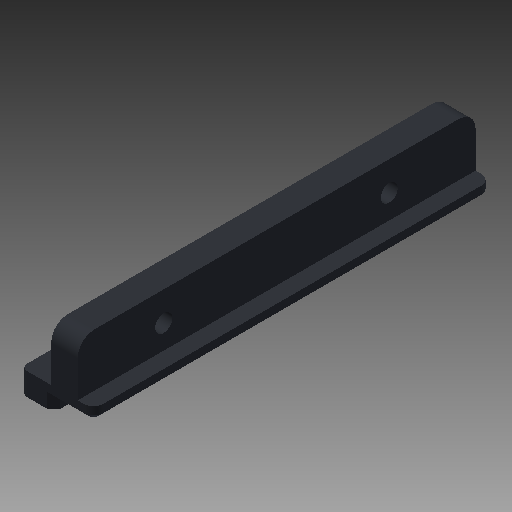
# Autodesk Inventor part: J007812
Saved by Autodesk Inventor 2018.3 (Build 223284000, 284)
## iProperties
Created: 2015-12-21
Material: VERO BLACK
Vendor: HHMI: JRC - ID&F
Document SubType Name: Modeling
Designer: ARNOLDJ
Density: 1.17 g/cm^3
Appearance: Black Anodize
Mass: 8.45789 g
Surface Area: 45.9199 cm^2
Volume: 7.22896 cm^3
Description: NRB LOW GUIDE RAIL INSERTS
Project: COMMON
Part Number: J007812
RuleStatus: InUse
AfterDocSave0: file://Part Number Cleaner
LAB/DEPT: COMMON
REQUESTING SCIENTIST: COMMON
SURFACE ROUGHNESS: N/A
DESIGN DEPARTMENT: HHMI: JRC - ID&F
SPECIAL FINISH: NONE
ALTERED ITEM PART NUMBER: N/A
ALTERED ITEM VENDOR: N/A
ALTERED ITEM DESCRIPTION: N/A
Revision Number: 0
Autodesk Inventor part; units mm, degrees
ref_plane "YZ Plane" through (0, 0, 0) normal (1, 0, 0) x (0, 1, 0)
ref_plane "XZ Plane" through (0, 0, 0) normal (0, 1, 0) x (-1, 0, 0)
ref_plane "XY Plane" through (0, 0, 0) normal (0, 0, 1) x (1, 0, 0)
sketch "Sketch1" plane through (0, 0, 0) normal (0, 0, 1) x (1, 0, 0)
  line L0 (0, 17.3736) -> (0, -2.8956) projected
  line L1 (-5.334, 0) -> (14.224, 0) projected
  line L2 (3.81, 1.778) -> (-2.54, 1.778)
  line L3 (-2.54, 1.778) -> (-2.54, 0)
  line L4 (-2.54, 0) -> (3.81, 0)
  line L5 (3.81, 0) -> (3.81, 1.778)
  line L6 (3.81, 1.778) -> (11.43, 1.778)
  line L7 (11.43, 1.778) -> (11.43, 4.318)
  line L8 (11.43, 4.318) -> (-2.54, 4.318)
  line L9 (-2.54, 4.318) -> (-2.54, 1.778)
  line L10 (8.382, 4.318) -> (3.302, 4.318)
  line L11 (3.302, 4.318) -> (3.302, 14.478)
  line L12 (3.302, 14.478) -> (8.382, 14.478)
  line L13 (8.382, 14.478) -> (8.382, 4.318)
  point P0 (0, 0)
  point P1 (0, 0.635)
  dimension "d1" = 2.54
  dimension "d2" = 1.778
  dimension "d25" = 2.54
  dimension "d26" = 10.16
  dimension "d27" = 5.08
  dimension "d49" = 3.302
  dimension "d50" = 2.54
  dimension "d51" = 11.43
  dimension "d52" = 3.81
  constraints: 24 end point, 5 perpendicular, 4 parallel, 3 horizontal, 3 point on line
  measures "d1" distance of L6.end L7.end
  measures "d2" distance of L4.end L2.start
  measures "d25" distance between parallel lines of L3 L0
  measures "d26" distance of L12.end L10.start
  measures "d27" distance of L11.end L12.end
  measures "d49" distance between parallel lines of L0 L11
  measures "d50" distance between parallel lines of L0 L9
  measures "d51" distance between parallel lines of L7 L0
  measures "d52" distance between parallel lines of L0 L5
extrude "Extrusion1" add sketch "Sketch1" along normal mid plane 76.2
sketch "Sketch2" plane through (-2.54, 4.318, 38.1) normal (0, 1, 0) x (1, 0, 0)
  line L0 (13.97, 76.2) -> (13.97, 0) projected
  line L1 (0, 76.2) -> (13.97, 76.2) projected
  line L2 (13.97, 0) -> (0, 0) projected
  line L3 (0, 76.2) -> (0, 0)
  line L4 (16.764, 38.1) -> (-2.794, 38.1) projected
  point P0 (2.54, 38.1)
  point P1 (2.54, 68.58)
  point P2 (2.54, 38.1)
  point P3 (2.54, 7.62)
  dimension "d6" = 30.48
  dimension "d7" = 30.48
  dimension "d48" = 2.54
  constraints: 2 end point, 2 vertical alignment, 1 coincident, 1 point on line
  measures "d6" distance of point (2.54, 38.1) point (2.54, 68.58)
  measures "d7" distance of point (2.54, 7.62) point (2.54, 38.1)
  measures "d48" distance from line of L3 point (2.54, 38.1)
hole "Hole1" at (0, 4.318, -30.48) at (0, 4.318, 30.48) direction (0, -1, 0) diameter 3.175 end through all
fillet "Fillet4" radius 1.905 2 edges at (11.43, 3.048, 38.1) (11.43, 3.048, -38.1)
chamfer "Chamfer4" distance 1.016 angle 45 5 edges at (11.43, 1.778, 0) (10.872, 1.778, 37.542) (6.6675, 1.778, 38.1) (10.872, 1.778, -37.542) (6.6675, 1.778, -38.1)
chamfer "Chamfer1" distance 1.27 angle 45 2 edges at (3.81, 0.889, 38.1) (3.81, 0.889, -38.1)
fillet "Fillet3" radius 1.27 2 edges at (-2.54, 2.159, -38.1) (-2.54, 2.159, 38.1)
fillet "Fillet5" radius 3.175 2 edges at (5.842, 14.478, 38.1) (5.842, 14.478, -38.1)
sketch "Sketch3" plane through (8.382, 4.318, 38.1) normal (1, 0, 0) x (0, 0, -1)
  line L0 (74.93, -4.318) -> (1.27, -4.318) projected
  line L1 (38.1, -7.2136) -> (38.1, 13.0556) projected
  point P0 (38.1, -4.318)
  point P1 (16.51, 4.572)
  point P2 (59.69, 4.572)
  dimension "d38" = 43.18
  dimension "d39" = 21.59
  dimension "d40" = 8.89
  measures "d38" distance of point (59.69, 4.572) point (16.51, 4.572)
  measures "d39" distance from line of L1 point (16.51, 4.572)
  measures "d40" distance from line of point (16.51, 4.572) L0
hole "Hole2" at (8.382, 8.89, 21.59) at (8.382, 8.89, -21.59) direction (-1, 0, 0) diameter 3.302 end through all
equation "\"d39\" = 0.5 * d38"
body "Solid1"
